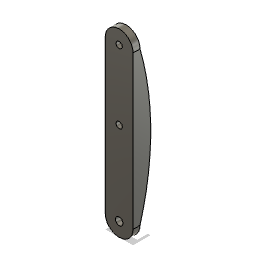
LRS_Holder v2 (Autodesk Fusion 360 design; units mm, degrees)
Autodesk Fusion 360 part; units mm, degrees
sketch "Skizze1" plane through (0, 0, 0) normal (0, 0, 1) x (1, 0, 0)
  circle A0 centre (0, 0) radius 2.25
  circle A1 centre (0, 50) radius 2.25
  circle A2 centre (0, -60) radius 2.75
  line L0 (0, 50) -> (0, 0)
  line L1 (0, 0) -> (0, -60)
  line L2 (-10, 50) -> (-10, -60)
  arc A3 (-10, -60) -> (10, -60) centre (0, -60) ccw
  line L3 (10, -60) -> (10, 50)
  arc A4 (10, 50) -> (-10, 50) centre (0, 50) ccw
  line L4 (0, 50) -> (0, -60) construction
  dimension "d1" = 5.5
  dimension "d2" = 4.5
  dimension "d3" = 50
  dimension "d4" = 60
  dimension "d5" = 10
  constraint coincident A0.centre L0.end
  constraint coincident A1.centre L0.start
  constraint vertical L0
  constraint coincident A2.centre L1.end
  constraint parallel L0 L1
  constraint equal A0 A1
  constraint tangent L2 A3
  constraint tangent A3 L3
  constraint parallel L2 L3
  constraint tangent L3 A4
  constraint tangent L2 A4
  constraint parallel L1 L4
  measures "d1" diameter of A2
  measures "d2" diameter of A1
  measures "d3" distance of A1.centre A0.centre
  measures "d4" distance of A0.centre A2.centre
  measures "d5" radius of A3
extrude "Extrusion1" add sketch "Skizze1" along normal blind 5 makes body 1
sketch "Skizze2" plane through (10, 0, 0) normal (1, 0, 0) x (0, 0, -1)
  line L0 (0, -60) -> (0, 50)
  line L1 (0, 50) -> (-5, 50)
  line L2 (-5, 50) -> (-5, -60)
  line L3 (-5, -60) -> (0, -60)
  circle A0 centre (-192.2888, -5) radius 200
  dimension "d8" = 400
  constraint coincident L0.end A0
  constraint coincident L0.start A0
  measures "d8" diameter of A0
extrude "Extrusion2" add sketch "Skizze2" against normal blind 2 contours L0 A0 bodies 1
split "Teilen1" by plane through (0, 0, 0) normal (1, 0, 0) bodies 1 makes body 2 at (3.9565, 33.3333, 5)
mirror "Spiegeln1" about plane through (0, 0, 0) normal (1, 0, 0) of bodies 2 merged
hidden bodies 1
equation "d4 = 40 mm + 20 mm"
